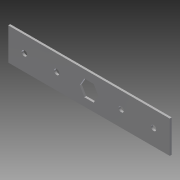
# Autodesk Inventor part: Steel Plate (0.0625)
Saved by Autodesk Inventor 2014 (Build 180170000, 170)
## iProperties
Created: 2014-01-12
Part Number: Steel Plate (0.0625)
Material: Steel
Document SubType Name: Modeling
Designer: Andrew Toennies
Mass: 37.7795 g
Surface Area: 67.0002 cm^2
Volume: 4.81267 cm^3
Density: 7.85 g/cm^3
Appearance: Steel
Author: Andrew Toennies
Autodesk Inventor part; units mm, degrees
ref_plane "YZ Plane" through (0, 0, 0) normal (1, 0, 0) x (0, 1, 0)
ref_plane "XZ Plane" through (0, 0, 0) normal (0, 1, 0) x (-1, 0, 0)
ref_plane "XY Plane" through (0, 0, 0) normal (0, 0, 1) x (1, 0, 0)
sketch "Sketch1" plane through (0, 0, 0) normal (0, 0, 1) x (1, 0, 0)
  line L0 (0, 0) -> (127, 0)
  line L1 (127, 0) -> (127, 25.4)
  line L2 (127, 25.4) -> (0, 25.4)
  line L3 (0, 25.4) -> (0, 0)
  line L4 (67.1662, 19.05) -> (70.8323, 12.7)
  line L5 (70.8323, 12.7) -> (67.1662, 6.35)
  line L6 (67.1662, 6.35) -> (59.8338, 6.35)
  line L7 (59.8338, 6.35) -> (56.1677, 12.7)
  line L8 (56.1677, 12.7) -> (59.8338, 19.05)
  line L9 (59.8338, 19.05) -> (67.1662, 19.05)
  circle A0 centre (12.7, 12.7) radius 2.0828
  circle A1 centre (114.3, 12.7) radius 2.0828
  circle A2 centre (88.9, 12.7) radius 2.0828
  circle A3 centre (38.1, 12.7) radius 2.0828
  point P0 (63.5, 12.7)
  dimension "d0" = 127
  dimension "d1" = 25.4
  dimension "d4" = 12.7
  dimension "d5" = 12.7
  dimension "d6" = 63.5
  dimension "d7" = 4.1656
  dimension "d8" = 4.1656
  dimension "d9" = 12.7
  dimension "d10" = 12.7
  dimension "d11" = 12.7
  dimension "d12" = 12.7
  dimension "d15" = 25.4
  dimension "d22" = 25.4
  constraints: 20 end point, 4 centre point, 4 horizontal, 2 parallel, 1 perpendicular, 17 other
  measures "d0" distance of L1.end L2.end
  measures "d1" distance of L0.end L1.end
  measures "d4" distance between parallel lines of L6 L9
  measures "d5" distance from line of L0 point (63.5, 12.7)
  measures "d6" distance from line of L1 point (63.5, 12.7)
  measures "d7" diameter of A0
  measures "d8" diameter of A1
  measures "d9" distance from line of L3 A0.centre
  measures "d10" distance from line of L0 A0.centre
  measures "d11" distance from line of L1 A1.centre
  measures "d12" distance from line of L0 A1.centre
  measures "d15" distance of A1.centre A2.centre
  measures "d22" distance of A0.centre A3.centre
extrude "Extrusion1" add sketch "Sketch1" along normal blind 1.5875
body "Solid1"
